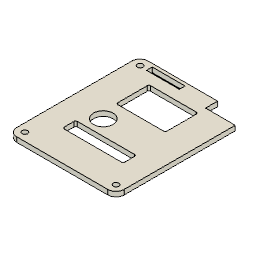
Mini Arcade Game Bottom (Autodesk Fusion 360 design; units mm, degrees)
part number: 2026-03-19-11-16-55-679
Autodesk Fusion 360 part; units mm, degrees
sketch "Sketch1" plane through (0, 0, 0) normal (0, 1, 0) x (1, 0, 0)
  line L0 (0, 0) -> (65.7, 0)
  line L1 (65.7, 0) -> (65.7, 80.4)
  line L2 (65.7, 80.4) -> (0, 80.4)
  line L3 (0, 80.4) -> (0, 0)
  circle A0 centre (5, 5) radius 1.7
  circle A1 centre (60.7, 5) radius 1.7
  circle A2 centre (5, 75.4) radius 1.7
  line L4 (65.7, 80.4) -> (47.5, 80.4)
  line L5 (47.5, 80.4) -> (47.5, 73)
  line L6 (47.5, 73) -> (65.7, 73)
  line L7 (65.7, 73) -> (65.7, 80.4)
  line L8 (9.5, 78.4) -> (29.5, 78.4)
  line L9 (29.5, 78.4) -> (29.5, 74.9)
  line L10 (29.5, 74.9) -> (9.5, 74.9)
  line L11 (9.5, 74.9) -> (9.5, 78.4)
  line L12 (14.35, 26.7) -> (51.35, 26.7)
  line L13 (51.35, 26.7) -> (51.35, 18.7)
  line L14 (51.35, 18.7) -> (14.35, 18.7)
  line L15 (14.35, 18.7) -> (14.35, 26.7)
  line L16 (17.85, 68) -> (47.85, 68)
  line L17 (47.85, 68) -> (47.85, 48)
  line L18 (47.85, 48) -> (17.85, 48)
  line L19 (17.85, 48) -> (17.85, 68)
  circle A3 centre (21.91, 36.02) radius 6
  dimension "d1" = 65.7
  dimension "d2" = 80.4
  dimension "d3" = 3.4
  dimension "d4" = 5
  dimension "d5" = 5
  dimension "d7" = 3.4
  dimension "d8" = 5
  dimension "d9" = 5
  dimension "d11" = 3.4
  dimension "d12" = 5
  dimension "d13" = 5
  dimension "d15" = 18.2
  dimension "d16" = 7.4
  dimension "d17" = 20
  dimension "d18" = 3.5
  dimension "d19" = 2
  dimension "d20" = 9.5
  dimension "d27" = 37
  dimension "d28" = 8
  dimension "d30" = 30
  dimension "d31" = 20
  dimension "d34" = 12
  dimension "d36" = 9.32
  dimension "d43" = 17.85
  constraint horizontal L0
  constraint vertical L1
  constraint horizontal L2
  constraint vertical L3
  constraint coincident L0.start L3.end
  constraint horizontal L4
  constraint vertical L5
  constraint horizontal L6
  constraint vertical L7
  constraint horizontal L8
  constraint vertical L9
  constraint horizontal L10
  constraint vertical L11
  constraint horizontal L12
  constraint vertical L13
  constraint horizontal L14
  constraint vertical L15
  constraint horizontal L16
  constraint vertical L17
  constraint horizontal L18
  constraint vertical L19
  measures "d1" distance of L0.start L0.end
  measures "d2" distance of L0.start L2.end
  measures "d3" diameter of A0
  measures "d4" distance of L0 A0.centre
  measures "d5" distance of L3 A0.centre
  measures "d7" diameter of A1
  measures "d8" distance of L0 A1.centre
  measures "d9" distance of L1 A1.centre
  measures "d11" diameter of A2
  measures "d12" distance of L2 A2.centre
  measures "d13" distance of L3 A2.centre
  measures "d15" distance of L1.end L4.end
  measures "d16" distance of L1.end L6.end
  measures "d17" distance of L8.start L8.end
  measures "d18" distance of L8.start L10.end
  measures "d19" distance of L2 L8
  measures "d20" distance of L3 L11
  measures "d27" distance of L12.start L12.end
  measures "d28" distance of L12.start L14.end
  measures "d30" distance of L16.start L16.end
  measures "d31" distance of L16.start L18.end
  measures "d34" diameter of A3
  measures "d36" distance of L12 A3.centre
  measures "d43" distance of L3 L19
extrude "Extrude1" add sketch "Sketch1" along normal blind 3 contours L0 L1 L2 L3 L5 L6
fillet "Fillet1" radius 5 3 edges at (65.7, 1.5, 0) (0, 1.5, 0) (0, 1.5, -80.4)
fillet "Fillet2" radius 1 8 edges at (17.85, 1.5, -68) (14.35, 1.5, -26.7) (47.85, 1.5, -68) (51.35, 1.5, -26.7) (51.35, 1.5, -18.7) (47.85, 1.5, -48) (17.85, 1.5, -48) (14.35, 1.5, -18.7)
